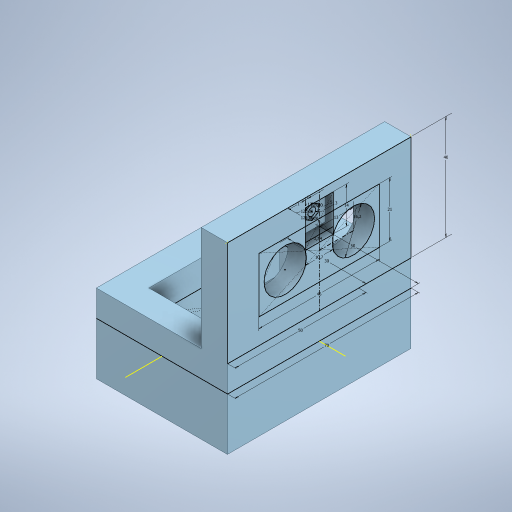
# Autodesk Inventor part: uMule-UDaR-sensor
Saved by Autodesk Inventor 2024.2 (Build 282272000, 272)
## iProperties
Created: 2009-02-10
Part Number: uMule-UDaR-sensor
Material: Ogólny
Document SubType Name: Modeling
Designer: owozn
Density: 1 g/cm^3
Appearance: Domyślna
Author: owozn
Autodesk Inventor part; units mm, degrees
ref_plane "YZ Plane" through (0, 0, 0) normal (1, 0, 0) x (0, 1, 0)
ref_plane "XZ Plane" through (0, 0, 0) normal (0, 1, 0) x (-1, 0, 0)
ref_plane "XY Plane" through (0, 0, 0) normal (0, 0, 1) x (1, 0, 0)
sketch "Szkic7" plane through (0, 0, 0) normal (0, 1, 0) x (-1, 0, 0)
  line L0 (0, -49) -> (0, 49) projected
  line L1 (35, 0) -> (-35, 0) projected
  line L2 (15, 25) -> (-15, 25)
  line L3 (-15, 25) -> (-15, -25)
  line L4 (-15, -25) -> (15, -25)
  line L5 (15, -25) -> (15, 25)
  line L6 (15, 25) -> (-15, -25) construction
  line L7 (-15, 25) -> (15, -25) construction
  line L8 (25, 35) -> (-25, 35)
  line L9 (-25, 35) -> (-25, -35)
  line L10 (-25, -35) -> (25, -35)
  line L11 (25, -35) -> (25, 35)
  line L12 (25, 35) -> (-25, -35) construction
  line L13 (-25, 35) -> (25, -35) construction
  line L14 (-15, 25) -> (-15, 35)
  line L15 (-15, -25) -> (-15, -35)
  point P0 (0, 0)
  dimension "d40" = 30
  dimension "d41" = 50
  dimension "d42" = 50
  dimension "d43" = 70
  constraints: 28 end point, 4 midpoint, 4 parallel, 3 perpendicular, 3 point on line, 2 horizontal
  measures "d40" distance of L4.end L3.end
  measures "d41" distance of L3.end L2.end
  measures "d42" distance of L10.end L9.end
  measures "d43" distance of L9.end L8.end
extrude "Wyciągnięcie proste6" add sketch "Szkic7" along normal blind 10 contours L10 L15 L4 L0 | L0 L4 L5 L1 L11 L10 | L10 L9 L1 L3 L15 | L1 L5 L2 L0 L8 L11 | L2 L14 L8 L0 | L1 L9 L8 L14 L3
extrude "Wyciągnięcie proste7" add sketch "Szkic7" along normal blind 50 contours L10 L9 L1 L3 L15 | L1 L9 L8 L14 L3
sketch "Szkic8" plane through (25, 0, 35) normal (1, 0, 0) x (0, 0, -1)
  line L0 (0, 10) -> (70, 10)
  line L1 (70, 10) -> (70, 50)
  line L2 (70, 50) -> (0, 50)
  line L3 (0, 50) -> (0, 10)
  line L4 (35, 50) -> (35, 10)
  circle A0 centre (48, 30) radius 8.1
  line L5 (48, 30) -> (35, 30)
  circle A1 centre (22, 30) radius 8.1
  line L6 (29.65, 46.662236) -> (40.35, 46.662236)
  line L7 (40.35, 46.662236) -> (40.35, 32.662236)
  line L8 (40.35, 32.662236) -> (29.65, 32.662236)
  line L9 (29.65, 32.662236) -> (29.65, 46.662236)
  line L10 (29.65, 46.662236) -> (40.35, 32.662236) construction
  line L11 (40.35, 46.662236) -> (29.65, 32.662236) construction
  circle A2 centre (32.15, 44.162236) radius 1.5
  line L12 (29.65, 44.162236) -> (30.65, 44.162236) construction
  line L13 (32.15, 46.662236) -> (32.15, 45.662236) construction
  line L14 (35, 32.662236) -> (35, 35.202236)
  line L15 (35, 35.202236) -> (40.35, 35.202236)
  line L16 (35, 35.202236) -> (29.65, 35.202236)
  circle A3 centre (32.15, 44.162236) radius 2.5 construction
  line L17 (29.65, 42.71886) -> (32.15, 41.275485)
  line L18 (32.15, 41.275485) -> (34.65, 42.71886)
  line L19 (29.65, 42.71886) -> (29.65, 45.605612)
  line L20 (29.65, 45.605612) -> (32.15, 47.048987)
  line L21 (32.15, 47.048987) -> (34.65, 45.605612)
  line L22 (34.65, 45.605612) -> (34.65, 42.71886)
  line L23 (12, 40.5) -> (58, 40.5)
  line L24 (58, 40.5) -> (58, 19.5)
  line L25 (58, 19.5) -> (12, 19.5)
  line L26 (12, 19.5) -> (12, 40.5)
  line L27 (12, 40.5) -> (58, 19.5) construction
  line L28 (58, 40.5) -> (12, 19.5) construction
  point P0 (35, 39.662236)
  point P1 (9.59459, 19.012494)
  point P2 (9.59459, 19.012494)
  point P3 (12.764463, 33.012494)
  point P4 (11.424717, 33.012494)
  point P5 (9.59459, 29.069118)
  point P6 (32.819873, 46.662236)
  point P7 (31.480127, 46.662236)
  dimension "d62" = 16.2
  dimension "d63" = 13
  dimension "d64" = 10.7
  dimension "d65" = 14
  dimension "d66" = 3
  dimension "d67" = 1
  dimension "d68" = 1
  dimension "d69" = 2.54
  dimension "d70" = 5
  dimension "d71" = 120
  dimension "d72" = 120
  dimension "d73" = 120
  dimension "d74" = 120
  dimension "d75" = 120
  dimension "d76" = 40
  dimension "d77" = 46
  dimension "d78" = 21
  constraints: 58 end point, 10 point on line, 8 midpoint, 6 parallel, 6 tangent, 5 perpendicular, 4 horizontal, 3 centre point, 3 coincident, 2 point on circle, 1 symmetric about line, 1 vertical, 4 other
  measures "d63" distance of L5.end L5.start
  measures "d64" distance of L7.end L8.end
  measures "d65" distance of L6.end L7.end
  measures "d66" diameter of A2
  measures "d67" distance of L12.start L12.end
  measures "d68" distance of L13.start L13.end
  measures "d69" distance of L14.start L14.end
  measures "d70" diameter of A3
  measures "d71" angle of L18 L17
  measures "d72" angle of L19 L17
  measures "d73" angle of L20 L19
  measures "d74" angle of L21 L20
  measures "d75" angle of L22 L21
  measures "d76" distance of L0.end L1.end
  measures "d77" distance of L24.end L25.end
  measures "d78" distance of L23.end L24.end
extrude "Wyciągnięcie proste8" cut sketch "Szkic8" against normal through all contours A1 | L25 L26 L23 L9 L8 L4 | L4 L5 A0 L7 L23 L24 L25 | L4 L8 A0 L5 | L8 L9 L16 L4 | L4 L15 L7 L8 | A0 | L23 L7 L15 L4 | L4 L16 L9 L23 | L21 L22 L18 L17 L9 L20 L6 | L6 L20 L21 | A2
extrude "Wyciągnięcie proste9" add sketch "Szkic8" against normal blind 7 contours L25 L26 L23 L9 L8 L4 | L4 L5 A0 L7 L23 L24 L25 | L4 L8 A0 L5 | L23 L7 L15 L4 | L4 L16 L9 L23 | L21 L22 L18 L17 L9 L20 L6 | L6 L20 L21
extrude "Wyciągnięcie proste10" cut sketch "Szkic8" against normal blind 3 contours L6 L7 L23 L4 | L4 L23 L9 L17 L18 L22 L21 L6 | L23 L7 L15 L4 | L4 L16 L9 L23 | L21 L22 L18 L17 L9 L20 L6 | L20 L9 L6
extrude "Wyciągnięcie proste11" add sketch "Szkic7" against normal blind 20 contours L10 L15 L4 L0 | L0 L4 L5 L1 L11 L10 | L10 L9 L1 L3 L15 | L1 L5 L2 L0 L8 L11 | L2 L14 L8 L0 | L1 L9 L8 L14 L3
